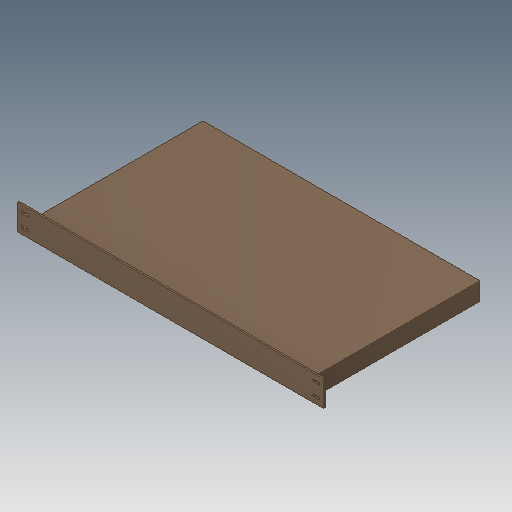
# Autodesk Inventor part: PatchPanel_rep
Saved by Autodesk Inventor 2017 (Build 210142000, 142)
## iProperties
Created: 2018-02-12
Part Number: PatchPanel_rep
Material: Generic
Document SubType Name: Modeling
Designer: Kathryn Rosie
Density: 1 g/cm^3
Appearance: Anodized - Bronze
Author: Kathryn Rosie
Autodesk Inventor part; units mm, degrees
ref_plane "YZ Plane" through (0, 0, 0) normal (1, 0, 0) x (0, 1, 0)
ref_plane "XZ Plane" through (0, 0, 0) normal (0, 1, 0) x (-1, 0, 0)
ref_plane "XY Plane" through (0, 0, 0) normal (0, 0, 1) x (1, 0, 0)
sketch "Sketch1" plane through (0, 0, 0) normal (0, 0, 1) x (1, 0, 0)
  line L0 (-241.3, -20.193) -> (241.3, -20.193)
  line L1 (241.3, -20.193) -> (241.3, 20.193)
  line L2 (241.3, 20.193) -> (-241.3, 20.193)
  line L3 (-241.3, 20.193) -> (-241.3, -20.193)
  line L4 (-241.3, -20.193) -> (241.3, 20.193) construction
  line L5 (241.3, -20.193) -> (-241.3, 20.193) construction
  point P0 (0, 0)
  dimension "d0" = 482.6
  dimension "d1" = 40.386
  constraints: 12 end point, 2 midpoint, 2 parallel, 1 horizontal, 1 perpendicular
  measures "d0" distance of L2.end L1.end
  measures "d1" distance of L1.end L0.end
extrude "Extrusion1" add sketch "Sketch1" against normal blind 2.6416
sketch "Sketch2" plane through (0, 0, -2.6416) normal (0, 0, -1) x (-1, 0, 0)
  line L0 (-241.3, -20.193) -> (241.3, -20.193) projected
  line L1 (-218.44, -20.193) -> (218.44, -20.193)
  line L2 (218.44, -20.193) -> (218.44, 7.913)
  line L3 (218.44, 7.913) -> (-218.44, 7.913)
  line L4 (-218.44, 7.913) -> (-218.44, -20.193)
  line L5 (0, -20.193) -> (0, 20.193) construction
  line L6 (241.3, 20.193) -> (-241.3, 20.193) projected
  point P0 (0, 0)
  dimension "d4" = 436.88
  constraints: 10 end point, 2 midpoint, 2 parallel, 1 horizontal, 1 perpendicular, 1 point on line, 1 other
  measures "d4" distance of L2.end L3.end
extrude "Extrusion2" add sketch "Sketch2" along normal blind 267.1064
sketch "Sketch3" plane through (0, 0, -2.6416) normal (0, 0, -1) x (-1, 0, 0)
  line L0 (-241.3, -20.193) -> (-218.44, -20.193) projected
  line L1 (-229.87, -20.193) -> (-229.87, 20.193) construction
  line L2 (229.87, -20.193) -> (229.87, 20.193) construction
  line L3 (241.3, -20.193) -> (241.3, 20.193) construction
  line L4 (241.3, 20.193) -> (-241.3, 20.193) construction
  line L5 (218.44, -20.193) -> (241.3, -20.193) construction
  line L6 (-233.6311, 10.0965) -> (-226.1089, 10.0965) construction
  line L7 (-233.6311, 7.939) -> (-226.1089, 7.939)
  line L8 (-226.1089, 12.254) -> (-233.6311, 12.254)
  arc A0 (-233.6311, 12.254) -> (-233.6311, 7.939) centre (-233.6311, 10.0965) ccw
  arc A1 (-226.1089, 7.939) -> (-226.1089, 12.254) centre (-226.1089, 10.0965) ccw
  line L9 (-241.3, 0) -> (241.3, 0) construction
  line L10 (-241.3, 20.193) -> (-241.3, -20.193) projected
  line L11 (-233.6311, -10.0965) -> (-226.1089, -10.0965) construction
  line L12 (-233.6311, -7.939) -> (-226.1089, -7.939)
  line L13 (-226.1089, -12.254) -> (-233.6311, -12.254)
  arc A2 (-233.6311, -7.939) -> (-233.6311, -12.254) centre (-233.6311, -10.0965) ccw
  arc A3 (-226.1089, -12.254) -> (-226.1089, -7.939) centre (-226.1089, -10.0965) ccw
  line L14 (0, 20.193) -> (0, -20.193) construction
  line L15 (-218.44, -20.193) -> (218.44, -20.193) projected
  line L16 (233.6311, 10.0965) -> (226.1089, 10.0965) construction
  line L17 (233.6311, 7.939) -> (226.1089, 7.939)
  line L18 (226.1089, 12.254) -> (233.6311, 12.254)
  arc A4 (233.6311, 7.939) -> (233.6311, 12.254) centre (233.6311, 10.0965) ccw
  arc A5 (226.1089, 12.254) -> (226.1089, 7.939) centre (226.1089, 10.0965) ccw
  arc A6 (226.1089, -7.939) -> (226.1089, -12.254) centre (226.1089, -10.0965) ccw
  line L19 (233.6311, -10.0965) -> (226.1089, -10.0965) construction
  line L20 (233.6311, -7.939) -> (226.1089, -7.939)
  line L21 (226.1089, -12.254) -> (233.6311, -12.254)
  arc A7 (233.6311, -12.254) -> (233.6311, -7.939) centre (233.6311, -10.0965) ccw
  point P0 (0, 0)
  point P1 (-229.87, 10.0965)
  point P2 (-229.87, -10.0965)
  point P3 (229.87, 10.0965)
  point P4 (229.87, -10.0965)
  dimension "d7" = 11.43
  dimension "d8" = 10.0965
  constraints: 40 end point, 21 symmetric about line, 16 point on circle, 8 centre point, 7 midpoint, 4 tangent, 3 point on line, 2 vertical, 1 parallel, 1 perpendicular, 6 other
  measures "d7" distance between parallel lines of L3 L2
  measures "d8" distance from line of L4 point (-229.87, 10.097)
extrude "Extrusion3" cut sketch "Sketch3" against normal up to surface (2.6416 mm away)
body "Solid1"
